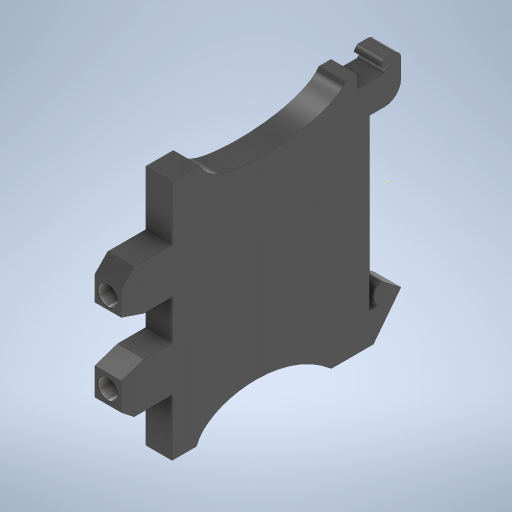
# Autodesk Inventor part: redna_stezaljka
Saved by Autodesk Inventor 2023 (Build 270158000, 158)
## iProperties
Created: 2022-07-15
Part Number: redna_stezaljka
Material: Generic
Document SubType Name: Sheet Metal
Designer: User
Density: 1 g/cm^3
Sheet Metal Rule: Default
Appearance: Default
Author: User
Autodesk Inventor part; units mm, degrees
ref_plane "YZ Plane" through (0, 0, 0) normal (1, 0, 0) x (0, 1, 0)
ref_plane "XZ Plane" through (0, 0, 0) normal (0, 1, 0) x (-1, 0, 0)
ref_plane "XY Plane" through (0, 0, 0) normal (0, 0, 1) x (1, 0, 0)
sketch "Sketch1" plane through (0, 0, 0) normal (0, 0, 1) x (1, 0, 0)
  point P0 (0, 0)
sketch "Sketch2" plane through (0, 0, 0) normal (0, 0, 1) x (1, 0, 0)
  line L0 (2.6, -23.75) -> (-2.6, -23.75)
  line L1 (-2.6, -23.75) -> (-2.6, 23.75)
  line L2 (-2.6, 23.75) -> (2.6, 23.75)
  line L3 (2.6, 23.75) -> (2.6, -23.75)
  line L4 (2.6, -23.75) -> (-2.6, 23.75) construction
  line L5 (-2.6, -23.75) -> (2.6, 23.75) construction
  point P0 (0, 0)
  dimension "d0" = 5.2
  dimension "d1" = 47.5
  constraints: 12 end point, 2 midpoint, 2 parallel, 1 horizontal, 1 perpendicular
  measures "d0" distance of L1.end L2.end
  measures "d1" distance of L2.end L0.start
extrude "Extrusion1" add sketch "Sketch2" along normal blind 45
sketch "Sketch3" plane through (0, 0, 45) normal (0, 0, 1) x (1, 0, 0)
  line L0 (-2.6, 23.75) -> (-2.6, -23.75) projected
  line L1 (2.6, 4.087) -> (-2.6, 4.087)
  line L2 (-2.6, 4.087) -> (-2.6, 12.977)
  line L3 (-2.6, 12.977) -> (2.6, 12.977)
  line L4 (2.6, 12.977) -> (2.6, 4.087)
  line L5 (2.6, 4.087) -> (-2.6, 12.977) construction
  line L6 (-2.6, 4.087) -> (2.6, 12.977) construction
  line L7 (2.6, -12.5814) -> (-2.6, -12.5814)
  line L8 (-2.6, -12.5814) -> (-2.6, -3.6914)
  line L9 (-2.6, -3.6914) -> (2.6, -3.6914)
  line L10 (2.6, -3.6914) -> (2.6, -12.5814)
  line L11 (2.6, -12.5814) -> (-2.6, -3.6914) construction
  line L12 (-2.6, -12.5814) -> (2.6, -3.6914) construction
  point P0 (0, 0)
  point P1 (0, 8.532)
  point P2 (0, -8.1364)
  dimension "d4" = 8.89
  dimension "d5" = 8.89
  constraints: 24 end point, 4 midpoint, 4 parallel, 2 horizontal, 2 perpendicular, 1 point on line
  measures "d4" distance of L9.end L7.start
  measures "d5" distance of L3.end L1.start
extrude "Extrusion2" add sketch "Sketch3" along normal blind 10
sketch "Sketch4" plane through (2.6, -23.75, 0) normal (1, 0, 0) x (0, 0, -1)
  line L0 (-55, 27.837) -> (-55, 36.727) projected
  line L1 (-55, 29.3595) -> (-50.526, 27.837)
  line L2 (-45, 27.837) -> (-55, 27.837) projected
  line L3 (-55, 20.0586) -> (-55, 11.1686) projected
  line L4 (-55, 18.5411) -> (-50.526, 20.0586)
  line L5 (-45, 20.0586) -> (-55, 20.0586) projected
  line L6 (-55, 34.1449) -> (-52.4593, 36.727)
  line L7 (-45, 36.727) -> (-55, 36.727) projected
  line L8 (-55, 13.172) -> (-52.4593, 11.1686)
  line L9 (-45, 11.1686) -> (-55, 11.1686) projected
  point P0 (0, 23.75)
  constraints: 8 end point, 8 point on line
extrude "Cut1" cut sketch "Sketch4" against normal blind 50
sketch "Sketch5" plane through (2.6, -23.75, 0) normal (1, 0, 0) x (0, 0, -1)
  line L0 (0, 0) -> (-45, 0) projected
  spline S0 degree 3 poles (-40.2107, 0) (-37.9135, 6.7697) (-18.8795, 9.6418) (-9.1773, -5.1937) knots 0 0 0 0 1 1 1 1
  line L1 (0, 47.5) -> (-45, 47.5) projected
  spline S1 degree 3 poles (-40.2107, 47.5) (-37.3937, 42.2325) (-16.5189, 40.6097) (-5.4427, 52.6048) knots 0 0 0 0 1 1 1 1
  spline S2 degree 4 poles (-5.4427, 52.6048) (-10.5459, 47.0782) (-1.7993, 73.7788) (-31.8751, 58.2429) (-24.9397, 58.0014) (-43.4335, 56.0468) (-40.2107, 47.9809) knots 0 0 0 0 0 0.322848 0.52405 1 1 1 1 1
  spline S3 degree 2 poles (-9.1773, -5.1937) (-32.7056, -23.415) (-40.2107, 0) knots 0 0 0 1 1 1
  point P0 (0, 23.75)
  point P1 (-36.1203, 3.965)
  point P2 (-24.7385, 5.2098)
  point P3 (-36.1203, 44.691)
  point P4 (-22.96, 43.8907)
  point P5 (-9.1773, 63.8088)
  point P6 (-21.8041, 62.5639)
  point P7 (-27.9396, 58.8292)
  point P8 (-35.5868, 55.9837)
  point P9 (-29.7915, -12.7663)
  constraints: 2 point on line, 17 other
extrude "Cut2" cut sketch "Sketch5" against normal blind 50 contours S0 S3 L0 | L0 S0
sketch "Sketch6" plane through (2.6, -23.75, 0) normal (1, 0, 0) x (0, 0, -1)
  line L0 (0, 47.5) -> (-45, 47.5) projected
  spline S0 degree 5 poles (-39.5697, 47.5) (-38.6935, 45.8855) (-36.3672, 43.6765) (-32.4153, 43.2932) (-19.2151, 40.9118) (4.5247, 51.2821) (-37.7534, 61.3423) (-41.4459, 53.794) (-40.6333, 49.4597) (-39.5697, 47.5) knots 0 0 0 0 0 0 0.205942 0.376454 0.576454 0.750023 1 1 1 1 1 1
  point P0 (0, 23.75)
  point P1 (-21.0742, 43.357)
  point P2 (-10.9372, 49.9371)
  point P3 (-38.9473, 54.1164)
  constraints: 1 point on line, 5 other
extrude "Cut3" cut sketch "Sketch6" against normal blind 50
sketch "Sketch7" plane through (2.6, -23.75, 0) normal (1, 0, 0) x (0, 0, -1)
  line L0 (0, 0) -> (-13.6901, 0) projected
  line L1 (-5.4242, 0) -> (0, 6.9885)
  line L2 (0, 0) -> (0, 47.5) projected
  line L3 (0, 6.9885) -> (-3.4745, 9.6852)
  spline S0 degree 4 poles (-3.4745, 9.6852) (-5.1889, 11.0158) (-7.9702, 5.5918) (-2.0544, 6.3) (-6.1809, 6.1911) knots 0 0 0 0 0 1 1 1 1 1
  line L4 (-6.1809, 6.1911) -> (-6.1809, 39.3557)
  line L5 (-6.1809, 39.3557) -> (2.94, 39.3545)
  line L6 (2.94, 39.3545) -> (2.9344, -5.3726)
  line L7 (2.9344, -5.3726) -> (-5.4248, -5.3715)
  line L8 (-5.4248, -5.3715) -> (-5.4242, 0)
  point P0 (0, 23.75)
  point P1 (-5.4511, 8.303)
  point P2 (-4.8217, 6.4274)
  constraints: 14 end point, 4 perpendicular, 2 point on line, 1 vertical, 5 other
extrude "Cut4" cut sketch "Sketch7" against normal blind 50
fillet "Fillet1" radius 3.175 1 edges at (0, 15.6049, 0)
fillet "Fillet2" radius 1.27 1 edges at (0, 23.75, 0)
sketch "Sketch8" plane through (2.6, -23.75, 45) normal (1, 0, 0) x (0, 0, -1)
  line L0 (43.73, 47.5) -> (34.0643, 47.5) projected
  line L1 (36.461, 47.5) -> (36.461, 45.1421)
  line L2 (36.461, 45.1421) -> (41.7089, 45.1421)
  spline S0 degree 4 poles (41.7089, 45.1421) (40.7946, 45.393) (48.2004, 47.9603) (38.2528, 44.519) (41.7089, 47.5) knots 0 0 0 0 0 1 1 1 1 1
  point P0 (45, 23.75)
  point P1 (42.4193, 45.7623)
  point P2 (43.1288, 46.2237)
  point P3 (41.7047, 46.2219)
  constraints: 4 end point, 2 point on line, 1 perpendicular, 1 vertical, 5 other
extrude "Cut5" cut sketch "Sketch8" against normal blind 50
sketch "Sketch9" plane through (0, 0, 55) normal (0, 0, 1) x (1, 0, 0)
  circle A0 centre (0, -7.8719) radius 1.905
  point P0 (0, 0)
  dimension "d21" = 3.81
  constraints: 1 centre point
  measures "d21" diameter of A0
extrude "Extrusion3" cut sketch "Sketch9" against normal blind 7
sketch "Sketch10" plane through (0, 0, 55) normal (0, 0, 1) x (1, 0, 0)
  circle A0 centre (0, 8.0498) radius 1.905
  point P0 (0, 0)
  dimension "d24" = 3.81
  constraints: 1 centre point
  measures "d24" diameter of A0
extrude "Extrusion4" cut sketch "Sketch10" against normal blind 7
equation "\"BendRadius\" = Thickness"
equation "\"BendReliefWidth\" = Thickness"
equation "\"BendReliefDepth\" = 0.5 * Thickness"
equation "\"CornerReliefSize\" = 4 * Thickness"
equation "\"MinimumRemnant\" = 2 * Thickness"
equation "\"TransitionRadius\" = BendRadius"
equation "\"JacobiRadiusSize\" = BendRadius"
equation "\"GapSize\" = Thickness"
equation "\"d8\" = Thickness"
equation "\"Thickness\" = 3.048"
body "Solid1"
